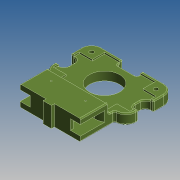
# Autodesk Inventor part: P123
Saved by Autodesk Inventor 2019 (Build 230136000, 136)
## iProperties
Created: 2016-10-17
Part Number: P123
Material: ABS Plastic
Document SubType Name: Modeling
Designer: serge.amoos
Density: 1.06 g/cm^3
Appearance: Olive Green
Mass: 52.3133 g
Surface Area: 167.275 cm^2
Volume: 49.3521 cm^3
Description: Charriot carré
Author: serge.amoos
Autodesk Inventor part; units mm, degrees
ref_plane "YZ Plane" through (0, 0, 0) normal (1, 0, 0) x (0, 1, 0)
ref_plane "XZ Plane" through (0, 0, 0) normal (0, 1, 0) x (-1, 0, 0)
ref_plane "XY Plane" through (0, 0, 0) normal (0, 0, 1) x (1, 0, 0)
sketch "Sketch1" plane through (0, 0, 0) normal (0, 0, 1) x (1, 0, 0)
  line L0 (-6, 0) -> (36, 0) construction
  line L1 (0, -30) -> (0, 5) construction
  line L2 (4.1, -22) -> (4.1, -25)
  line L3 (4.1, -25) -> (0, -25)
  line L4 (30, 0) -> (30, -22)
  line L5 (0, 0) -> (30, 0)
  line L6 (30, -22) -> (4.1, -22)
  line L7 (0, 0) -> (0, -25)
  point P0 (0, 0)
  dimension "d42" = 22
  dimension "d43" = 4.1
  dimension "d44" = 30
  dimension "d45" = 3
  constraints: 12 end point, 3 collinear, 2 point on line
  measures "d42" distance between parallel lines of L6 L0
  measures "d43" distance between parallel lines of L1 L2
  measures "d44" distance between parallel lines of L4 L1
  measures "d45" distance between parallel lines of L3 L6
extrude "Extrusion2" add sketch "Sketch1" along normal mid plane 20
sketch "Sketch3" plane through (0, 0, 0) normal (0, 0, 1) x (1, 0, 0)
  line L0 (30, -22) -> (4.1, -22) construction
  line L1 (4.1, -22) -> (4.1, -25) construction
  line L2 (4.1, -25) -> (0, -25) construction
  line L3 (0, 0) -> (30, 0) construction
  line L4 (-6, 0) -> (36, 0) construction
  line L5 (0, -56.4) -> (0, 9.4) construction
  arc A0 (14, -17) -> (19.2361, -19) centre (17, -17) ccw
  line L6 (14, -17) -> (14, 0)
  line L7 (14, 0) -> (30, 0)
  line L8 (20, -22) -> (20, -19)
  line L9 (30, -22) -> (30, 0)
  line L10 (0, -25) -> (0, 0) projected
  line L11 (30, 0) -> (30, -22) projected
  line L12 (19.2361, -19) -> (20, -19)
  line L13 (20, -22) -> (30, -22)
  point P0 (30, 0)
  point P1 (20, -47)
  dimension "d19" = 3
  dimension "d20" = 5
  dimension "d62" = 3
  dimension "d245" = 20
  dimension "d246" = 17
  constraints: 12 end point, 3 collinear, 2 point on circle, 1 centre point, 1 perpendicular, 1 point on line, 1 tangent, 1 vertical
  measures "d19" radius of A0
  measures "d20" distance from line of L0 A0.centre
  measures "d62" distance between parallel lines of L0 L12
  measures "d245" distance between parallel lines of L8 L5
  measures "d246" distance from line of L10 A0.centre
extrude "Extrusion3" cut sketch "Sketch3" along normal mid plane 10
sketch "Sketch6" plane through (0, -25, 10) normal (-1, 0, 0) x (0, 0, 1)
  line L0 (-10, -5) -> (-10, 30) projected
  line L1 (-24, 25) -> (4, 25) projected
  line L2 (-20, 0) -> (0, 0) projected
  point P0 (-10, 25)
  point P1 (-10, 21)
  dimension "d49" = 4
  constraints: 1 point on line
  measures "d49" distance from line of point (-10, 21) L1
hole "Trou pour ressort" at (0, -4, 0) direction (1, 0, 0) diameter 5 end through all
mirror "Mirror1" about plane through (0, 0, 0) normal (-1, 0, 0)
sketch "Sketch8" plane through (14, 0, 5) normal (0, 1, 0) x (1, 0, 0)
  line L0 (16, 10) -> (0, 10) construction
  line L1 (0, 10) -> (0, 0) construction
  line L2 (0, 0) -> (16, 0) construction
  line L3 (16, 0) -> (16, -5) construction
  line L4 (16, -5) -> (-44, -5) construction
  line L5 (-44, -5) -> (-44, 0) construction
  line L6 (-44, 0) -> (-28, 0) construction
  line L7 (-28, 0) -> (-28, 10) construction
  line L8 (-28, 10) -> (-44, 10) construction
  line L9 (-44, 10) -> (-44, 15) construction
  line L10 (-44, 15) -> (16, 15) construction
  line L11 (16, 15) -> (16, 10) construction
  line L12 (-44, -5) -> (16, -5)
  line L13 (16, -5) -> (16, 15)
  line L14 (16, 15) -> (-44, 15)
  line L15 (-44, 15) -> (-44, -5)
  point P0 (-14, 5)
  constraints: 8 end point, 2 parallel, 1 horizontal, 1 perpendicular
extrude "Extrusion5" add sketch "Sketch8" along normal blind 2
sketch "Sketch9" plane through (14, 2, 5) normal (0, 1, 0) x (1, 0, 0)
  line L0 (-44, 15) -> (16, 15) construction
  line L1 (16, 15) -> (16, -5) construction
  line L2 (16, -5) -> (-44, -5) construction
  line L3 (-44, -5) -> (-44, 15) construction
  line L4 (-44, 15) -> (16, 15)
  line L5 (16, 15) -> (16, -5)
  line L6 (16, -5) -> (-44, -5)
  line L7 (-44, -5) -> (-44, 15)
  line L8 (-14, 19) -> (-14, -9) construction
  line L9 (16, 15) -> (-44, 15) projected
  line L10 (-44, -5) -> (16, -5) projected
  line L11 (-44, 15) -> (-44, -5) projected
  line L12 (-44, 15) -> (-55, 15)
  line L13 (-55, 15) -> (-55, -5)
  line L14 (-55, -5) -> (-44, -5)
  line L15 (-44, -5) -> (-44, 15)
  line L16 (16, 15) -> (27, 15)
  line L17 (27, 15) -> (27, -5)
  line L18 (27, -5) -> (16, -5)
  line L19 (16, -5) -> (16, 15)
  point P0 (-14, 5)
  point P1 (-14, 15)
  dimension "d266" = 41
  dimension "d267" = 41
  constraints: 24 end point, 6 parallel, 4 collinear, 3 horizontal, 3 perpendicular, 2 point on line, 1 midpoint
  measures "d266" distance between parallel lines of L8 L13
  measures "d267" distance between parallel lines of L17 L8
extrude "Extrusion6" add sketch "Sketch9" along normal blind 58
fillet "Fillet3" radius 16 2 edges at (-30, 0, 0) (30, 0, 0)
sketch "Sketch12" plane through (-14, -17, -5) normal (-1, 0, 0) x (0, 0, 1)
  line L0 (5, -25) -> (5, 94) projected
  line L1 (15, -8) -> (-5, -8) projected
  point P0 (5, 17)
  point P1 (5, 3.5)
  dimension "d78" = 11.5
  constraints: 1 point on line
  measures "d78" distance from line of point (5, 3.5) L1
hole "Hole5" at (-14, -13.5, 0) direction (1, 0, 0) diameter 6 end through all
sketch "Sketch22" plane through (0, 0, 0) normal (1, 0, 0) x (0, 1, 0)
  line L0 (60, -10) -> (-25, -10) construction
  line L1 (-25, -10) -> (-25, 10) construction
  line L2 (-25, 10) -> (60, 10) construction
  circle A0 centre (-13.5, 0) radius 3 construction
  circle A1 centre (-4, 0) radius 2.5 construction
  line L3 (75.5267, 17.9704) -> (6, 17.9704)
  line L4 (6, 17.9704) -> (6, 0)
  line L5 (6, 0) -> (75.5267, 0)
  line L6 (75.5267, 0) -> (75.5267, 17.9704)
  line L7 (62, -10) -> (32, -10) projected
  line L8 (60, 10) -> (60, -10) projected
  point P0 (0, 0)
  dimension "d213" = 10
  constraints: 8 end point, 2 parallel, 1 horizontal, 1 perpendicular
  measures "d213" distance between parallel lines of L0 L5
extrude "Extrusion13" cut sketch "Sketch22" along normal through all both and the other way through all
sketch "Sketch29" plane through (0, 0, 10) normal (0, 0, 1) x (1, 0, 0)
  line L0 (57.4, -4) -> (-57.4, -4) projected
  line L1 (14, -10.5) -> (14, -16.5) projected
  line L2 (14, -1.5) -> (14, -6.5) projected
  line L3 (14, -17) -> (14, 0) projected
  line L4 (14, 0) -> (14, -17) projected
  point P0 (0, 0)
  point P1 (17, -4)
  dimension "d205" = 3
  constraints: 1 point on line
  measures "d205" distance from line of point (17, -4) L2
hole "Hole12" at (17, -4, 10) direction (0, 0, -1) diameter 1.5 depth 2 tip angle 118
mirror "Mirror4" about plane through (0, 0, 0) normal (1, 0, 0) of "Hole12"
sketch "Sketch36" plane through (-30, 60, 0) normal (0, 0, 1) x (1, 0, 0)
  line L0 (-27.4, -60) -> (87.4, -60) projected
  line L1 (30, -102) -> (30, 17) projected
  point P0 (30, -60)
  point P1 (30, -28)
  dimension "d258" = 32
  constraints: 1 point on line
  measures "d258" distance from line of point (30, -28) L0
hole "Hole16" at (0, 32, 0) direction (0, 0, -1) diameter 30 end through all
sketch "Sketch38" plane through (0, 0, 10) normal (0, 0, 1) x (1, 0, 0)
  line L0 (30, -22) -> (30, 2) construction
  line L1 (30, 2) -> (41, 2) construction
  line L2 (41, 60) -> (41, 6) construction
  line L3 (30, 2) -> (41, 2)
  line L4 (41, 2) -> (41, 12)
  line L5 (41, 12) -> (30, 12)
  line L6 (30, 12) -> (30, 2)
  line L7 (-57.4, 0) -> (57.4, 0) projected
  line L8 (0, -42) -> (0, 77) projected
  circle A0 centre (0, 32) radius 15 projected
  line L9 (-41, 2) -> (-30, 2) projected
  line L10 (-41, 6) -> (-41, 60) projected
  line L11 (-30, 2) -> (-41, 2)
  line L12 (-41, 2) -> (-41, 12)
  line L13 (-41, 12) -> (-30, 12)
  line L14 (-30, 12) -> (-30, 2)
  point P0 (0, 0)
  dimension "d272" = 20
  constraints: 16 end point, 4 parallel, 2 horizontal, 2 perpendicular, 2 point on line, 1 collinear
  measures "d272" distance from line of L5 A0.centre
extrude "Extrusion20" cut sketch "Sketch38" against normal through all contours L6 L5 L4 L3 | L12 L10 L13 L14 L9
fillet "Fillet30" radius 10 2 edges at (41, 12, -5) (-41, 12, -5)
fillet "Fillet31" radius 10 2 edges at (41, 60, -5) (-41, 60, -5)
sketch "Sketch39" plane through (-41, 6, 0) normal (0, 0, 1) x (1, 0, 0)
  circle A0 centre (41, 26) radius 15 construction
  line L0 (-16.4, -6) -> (98.4, -6) construction
  line L1 (41, -48) -> (41, 71) construction
  line L2 (79.1, 13) -> (2.9, 13)
  line L3 (2.9, 13) -> (2.9, 39)
  line L4 (2.9, 39) -> (79.1, 39)
  line L5 (79.1, 39) -> (79.1, 13)
  line L6 (66.25, 0.75) -> (15.75, 0.75)
  line L7 (15.75, 0.75) -> (15.75, 51.25)
  line L8 (15.75, 51.25) -> (66.25, 51.25)
  line L9 (66.25, 51.25) -> (66.25, 0.75)
  point P0 (41, -6)
  point P1 (41, 13)
  point P2 (2.9, 26)
  point P3 (41, 0.75)
  point P4 (15.75, 26)
  dimension "d277" = 76.2
  dimension "d278" = 26
  dimension "d281" = 50.5
  dimension "d282" = 50.5
  constraints: 16 end point, 4 midpoint, 4 parallel, 2 horizontal, 2 horizontal alignment, 2 perpendicular, 2 point on line
  measures "d277" distance of L2.start L2.end
  measures "d278" distance between parallel lines of L4 L2
  measures "d281" distance of L6.start L6.end
  measures "d282" distance of L8.end L6.start
extrude "Extrusion21" cut sketch "Sketch39" against normal blind 1.5
sketch "Sketch40" plane through (-30, 6, 0) normal (0, 0, 1) x (1, 0, 0)
  line L0 (-53.8568, -6) -> (104.5258, -6) construction
  line L1 (30, -48.4142) -> (30, 73.4853) construction
  circle A0 centre (30, 26) radius 15 construction
  line L2 (68.1, 13) -> (68.1, 39) construction
  line L3 (68.1, 39) -> (55.25, 39) construction
  line L4 (55.25, 39) -> (55.25, 51.25) construction
  line L5 (55.25, 51.25) -> (4.75, 51.25) construction
  line L6 (4.75, 51.25) -> (4.75, 39) construction
  line L7 (4.75, 39) -> (-8.1, 39) construction
  line L8 (-8.1, 39) -> (-8.1, 13) construction
  line L9 (-8.1, 13) -> (4.75, 13) construction
  line L10 (4.75, 13) -> (4.75, 0.75) construction
  line L11 (4.75, 0.75) -> (55.25, 0.75) construction
  line L12 (55.25, 0.75) -> (55.25, 13) construction
  line L13 (55.25, 13) -> (68.1, 13) construction
  line L14 (44, -16.5) -> (16, -16.5) construction
  line L15 (16, -16.5) -> (16, -12.5) construction
  line L16 (16, -12.5) -> (44, -12.5) construction
  line L17 (44, -12.5) -> (44, -16.5) construction
  arc A1 (0, -4) -> (7.746, -6) centre (7.746, 10) ccw construction
  line L18 (0, -4) -> (0, 0) construction
  line L19 (0, 0) -> (60, 0) construction
  line L20 (60, 6) -> (60, 0) construction
  line L21 (61, 6) -> (60, 6) construction
  arc A2 (61, 6) -> (71, 16) centre (61, 16) ccw construction
  line L22 (71, 44) -> (71, 16) construction
  arc A3 (71, 44) -> (61, 54) centre (61, 44) ccw construction
  line L23 (-1, 54) -> (61, 54) construction
  arc A4 (-1, 54) -> (-11, 44) centre (-1, 44) ccw construction
  line L24 (-11, 16) -> (-11, 44) construction
  arc A5 (-11, 16) -> (-1, 6) centre (-1, 16) ccw construction
  line L25 (0, 6) -> (-1, 6) construction
  line L26 (0, 0) -> (0, 6) construction
  line L27 (16, -6) -> (7.746, -6) construction
  line L28 (16, -7.5) -> (16, -6) construction
  line L29 (44, -7.5) -> (16, -7.5) construction
  line L30 (44, -6) -> (44, -7.5) construction
  line L31 (52.254, -6) -> (44, -6) construction
  arc A6 (52.254, -6) -> (60, -4) centre (52.254, 10) ccw construction
  line L32 (60, 0) -> (60, -4) construction
  line L33 (50, -25) -> (50, -28) construction
  line L34 (50, -28) -> (34.1, -28) construction
  line L35 (34.1, -28) -> (34.1, -31) construction
  line L36 (34.1, -31) -> (25.9, -31) projected
  line L37 (25.9, -31) -> (25.9, -28) construction
  line L38 (25.9, -28) -> (10, -28) construction
  line L39 (10, -28) -> (10, -25) construction
  line L40 (10, -25) -> (10.7639, -25) construction
  arc A7 (10.7639, -25) -> (16, -23) centre (13, -23) ccw construction
  line L41 (16, -23) -> (16, -22.5) construction
  line L42 (16, -22.5) -> (44, -22.5) construction
  line L43 (44, -22.5) -> (44, -23) construction
  arc A8 (44, -23) -> (49.2361, -25) centre (47, -23) ccw construction
  line L44 (49.2361, -25) -> (50, -25) construction
  line L45 (81.8997, 26) -> (-31.2307, 26) construction
  line L46 (71, 18.5) -> (63, 18.5)
  line L47 (63, 18.5) -> (63, 33.5)
  line L48 (63, 33.5) -> (71, 33.5)
  line L49 (71, 33.5) -> (71, 18.5)
  point P0 (30, -6)
  point P1 (63, 26)
  dimension "d283" = 8
  dimension "d284" = 15
  constraints: 10 end point, 3 point on line, 2 horizontal, 2 parallel, 1 midpoint, 1 perpendicular
  measures "d283" distance of L46.start L46.end
  measures "d284" distance of L46.end L47.end
extrude "Extrusion22" cut sketch "Sketch40" against normal through all
fillet "Fillet32" radius 1 2 edges at (41, 24.5, -5) (41, 39.5, -5)
fillet "Fillet33" radius 5 2 edges at (33, 24.5, -5.75) (33, 39.5, -5.75)
mirror "Mirror6" about plane through (0, 0, 0) normal (1, 0, 0) of "Extrusion22"
fillet "Fillet34" radius 5 2 edges at (-33, 24.5, -5.75) (-33, 39.5, -5.75)
fillet "Fillet35" radius 1 2 edges at (-41, 24.5, -5) (-41, 39.5, -5)
sketch "Sketch41" plane through (-31, 60, 0) normal (0, 0, 1) x (1, 0, 0)
  line L0 (-26.4, -60) -> (88.4, -60) construction
  line L1 (31, -102) -> (31, 17) construction
  line L2 (0, 0) -> (62, 0) construction
  line L3 (41, 0) -> (21, 0)
  line L4 (21, 0) -> (21, -6)
  line L5 (21, -6) -> (41, -6)
  line L6 (41, -6) -> (41, 0)
  point P0 (31, -60)
  point P1 (31, -6)
  dimension "d291" = 20
  dimension "d292" = 6
  constraints: 8 end point, 2 parallel, 1 collinear, 1 horizontal, 1 midpoint, 1 perpendicular, 1 point on line
  measures "d291" distance of L4.end L5.end
  measures "d292" distance between parallel lines of L2 L5
extrude "Extrusion23" cut sketch "Sketch41" against normal through all
fillet "Fillet36" radius 1 2 edges at (10, 60, -5) (-10, 60, -5)
fillet "Fillet37" radius 2 2 edges at (10, 54, -5.75) (-10, 54, -5.75)
fillet "Fillet38" radius 2 2 edges at (30, 12, -5) (-30, 12, -5)
fillet "Fillet39" radius 1 35 edges at (-30.528, 11.3957, -10) (-38.3598, 15.23, -10) (-41, 22.75, -10) (-41, 45.25, -10) (-40.7071, 24.2071, -10) (-39, 24.5, -10) (-34.4645, 25.9645, -10) (-33, 32, -10) (-34.4645, 38.0355, -10) (-39, 39.5, -10) (-40.7071, 39.7929, -10) (-38.0711, 57.0711, -10) (-21, 60, -10) (21, 60, -10) (-10.2929, 59.7071, -10) (-10, 57.5, -10) (-9.4142, 54.5858, -10) (0, 54, -10) (9.4142, 54.5858, -10) (10, 57.5, -10) (10.2929, 59.7071, -10) (38.0711, 57.0711, -10) (41, 22.75, -10) (41, 45.25, -10) (40.7071, 39.7929, -10) (39, 39.5, -10) (34.4645, 38.0355, -10) (33, 32, -10) (34.4645, 25.9645, -10) (39, 24.5, -10) (40.7071, 24.2071, -10) (38.3598, 15.23, -10) (30.528, 11.3957, -10) (30, -5.9791, -10) (-30, -5.9791, -10)
fillet "Fillet42" radius 1 15 edges at (34.4645, 38.0355, -1.5) (38.05, 39.5, -1.5) (34.4645, 25.9645, -1.5) (38.05, 24.5, -1.5) (33, 32, -1.5) (-33, 32, -1.5) (-34.4645, 38.0355, -1.5) (-38.05, 39.5, -1.5) (-38.05, 24.5, -1.5) (-34.4645, 25.9645, -1.5) (-9.4142, 54.5858, -1.5) (-10, 56.625, -1.5) (9.4142, 54.5858, -1.5) (10, 56.625, -1.5) (0, 54, -1.5)
sketch "Sketch43" plane through (-38.1, 45, 0) normal (0, 0, 1) x (1, 0, 0)
  line L0 (-19.3, -45) -> (95.5, -45) projected
  line L1 (38.1, -87) -> (38.1, 32) projected
  point P0 (38.1, -45)
  point P1 (6.1, 6)
  dimension "d304" = 32
  dimension "d305" = 51
  measures "d304" distance from line of L1 point (6.1, 6)
  measures "d305" distance from line of L0 point (6.1, 6)
hole "Hole17" at (-32, 51, 0) direction (0, 0, -1) diameter 4 end through all
mirror "Mirror7" about plane through (0, 0, 0) normal (1, 0, 0) of "Hole17"
fillet "Fillet43" radius 2 1 edges at (0, 6, 10)
fillet "Fillet45" radius 2 1 edges at (0, 6, 0)
fillet "Fillet46" radius 1 34 edges at (30, 5.4142, 9.4142) (30, 6, 5) (30, 6.5858, 0.5858) (30, 9.0209, 0) (30.528, 11.3957, 0) (38.3598, 15.23, 0) (41, 22.75, 0) (40.7071, 24.2071, 0) (39.05, 24.5, 0) (30, -9, 10) (40.7071, 39.7929, 0) (39.05, 39.5, 0) (38.0711, 57.0711, 0) (21, 60, 0) (10.2929, 59.7071, 0) (10, 58.125, 0) (41, 45.25, 0) (-10.2929, 59.7071, 0) (-10, 58.125, 0) (-38.0711, 57.0711, 0) (-41, 45.25, 0) (-40.7071, 39.7929, 0) (-39.05, 39.5, 0) (-21, 60, 0) (-41, 22.75, 0) (-40.7071, 24.2071, 0) (-39.05, 24.5, 0) (-30.528, 11.3957, 0) (-30, 9.0209, 0) (-30, 6.5858, 0.5858) (-30, 6, 5) (-30, 5.4142, 9.4142) (-30, -9, 10) (-38.3598, 15.23, 0)
body "Solid2"
